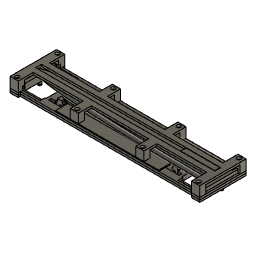
Switch blade (Autodesk Fusion 360 design; units mm, degrees)
Autodesk Fusion 360 part; units mm, degrees
note: some values were not read from the file. Chosen so that the rebuilt part matches the saved one: which bodies a step acts on; which face or edge a step refers to. Set by a fixed rule: which sketch regions a step uses.
(part 1 of 2)
sketch "base" plane through (0, 0, 0) normal (0, 0, 1) x (1, 0, 0)
  line L0 (0, 0) -> (180, 0)
  line L1 (180, 0) -> (180, 40)
  line L2 (180, 40) -> (0, 40)
  line L3 (0, 40) -> (0, 0)
  dimension "d3" = 40
  dimension "d4" = 180
  constraint horizontal L0
  constraint vertical L1
  constraint horizontal L2
  constraint vertical L3
  constraint coincident L0.start L3.end
  measures "d3" distance of L0.start L2.end
  measures "d4" distance of L0.start L0.end
ref_plane "WorkPlane1" through (90, 20, 2) normal (0, 0, 1) x (1, 0, 0)
sketch "catchCutout" plane through (0, 0, 2) normal (0, 0, 1) x (1, 0, 0)
  line L0 (147.75, 33.25) -> (144.75, 33.25)
  line L1 (144.75, 33.25) -> (144.75, 10)
  line L2 (144.75, 10) -> (147.75, 10)
  line L3 (147.75, 10) -> (147.75, 33.25)
  line L4 (144.5, 33.5) -> (148, 33.5)
  line L5 (148, 33.5) -> (148, 6.5)
  line L6 (148, 6.5) -> (144.5, 6.5)
  line L7 (144.5, 6.5) -> (144.5, 33.5)
  line L8 (150, 0) -> (150, 40)
  line L9 (0, 0) -> (150, 0)
  line L10 (150, 40) -> (0, 40)
  line L11 (144.75, 10) -> (141.75, 10)
  line L12 (141.75, 10) -> (141.75, 14)
  line L13 (141.75, 14) -> (144.75, 14)
  line L14 (144.75, 14) -> (144.75, 10)
  line L15 (144.5, 6.5) -> (125.5, 6.5)
  line L16 (125.5, 6.5) -> (125.5, 14.25)
  line L17 (125.5, 14.25) -> (144.5, 14.25)
  line L18 (144.5, 14.25) -> (144.5, 6.5)
  circle A0 centre (128.5, 9.5) radius 2.5
  line L19 (90, 40) -> (90, 0)
  line L20 (144.5, 18.0289) -> (148, 18.0289)
  line L21 (147.75, 10) -> (151.75, 10)
  line L22 (151.75, 10) -> (151.75, 12)
  line L23 (151.75, 12) -> (147.75, 12)
  line L24 (147.75, 12) -> (147.75, 10)
  line L25 (148, 6.5) -> (152, 6.5)
  line L26 (152, 6.5) -> (152, 9)
  line L27 (152, 9) -> (148, 9)
  line L28 (148, 9) -> (148, 6.5)
  line L29 (152, 9) -> (148, 9)
  line L30 (148, 9) -> (148, 12.25)
  line L31 (148, 12.25) -> (152, 12.25)
  line L32 (152, 12.25) -> (152, 9)
  line L33 (144.75, 33.25) -> (140.75, 33.25)
  line L34 (140.75, 33.25) -> (140.75, 31.25)
  line L35 (140.75, 31.25) -> (144.75, 31.25)
  line L36 (144.75, 31.25) -> (144.75, 33.25)
  line L37 (144.5, 33.5) -> (140.5, 33.5)
  line L38 (140.5, 33.5) -> (140.5, 30.25)
  line L39 (140.5, 30.25) -> (144.5, 30.25)
  line L40 (144.5, 30.25) -> (144.5, 33.5)
  line L41 (140.5, 30.25) -> (144.5, 30.25)
  line L42 (144.5, 30.25) -> (144.5, 27.75)
  line L43 (144.5, 27.75) -> (140.5, 27.75)
  line L44 (140.5, 27.75) -> (140.5, 30.25)
  line L45 (147.75, 12) -> (139.7117, 12)
  line L46 (144.5, 27.75) -> (148, 27.75)
  line L47 (144.75, 31.25) -> (147.75, 31.25)
  line L48 (35.25, 31.25) -> (35.25, 33.25)
  line L49 (28, 12.25) -> (28, 9)
  line L50 (39.5, 27.75) -> (39.5, 30.25)
  line L51 (32.25, 10) -> (28.25, 10)
  line L52 (35.5, 18.0289) -> (32, 18.0289)
  line L53 (38.25, 10) -> (38.25, 14)
  line L54 (35.25, 33.25) -> (35.25, 10)
  line L55 (32.25, 10) -> (32.25, 33.25)
  line L56 (35.5, 6.5) -> (35.5, 33.5)
  line L57 (28.25, 10) -> (28.25, 12)
  line L58 (32, 12.25) -> (28, 12.25)
  line L59 (38.25, 14) -> (35.25, 14)
  line L60 (54.5, 14.25) -> (35.5, 14.25)
  line L61 (32, 9) -> (32, 12.25)
  circle A1 centre (51.5, 9.5) radius 2.5
  line L62 (28.25, 12) -> (32.25, 12)
  line L63 (32, 33.5) -> (32, 6.5)
  line L64 (32.25, 12) -> (40.2883, 12)
  line L65 (28, 6.5) -> (28, 9)
  line L66 (35.25, 10) -> (32.25, 10)
  line L67 (35.25, 14) -> (35.25, 10)
  line L68 (32, 6.5) -> (35.5, 6.5)
  line L69 (35.25, 33.25) -> (39.25, 33.25)
  line L70 (32, 9) -> (32, 6.5)
  line L71 (35.5, 27.75) -> (32, 27.75)
  line L72 (35.25, 10) -> (38.25, 10)
  line L73 (28, 9) -> (32, 9)
  line L74 (39.25, 33.25) -> (39.25, 31.25)
  line L75 (32.25, 12) -> (32.25, 10)
  line L76 (35.5, 33.5) -> (39.5, 33.5)
  line L77 (39.25, 31.25) -> (35.25, 31.25)
  line L78 (32.25, 33.25) -> (35.25, 33.25)
  line L79 (35.5, 27.75) -> (39.5, 27.75)
  line L80 (39.5, 30.25) -> (35.5, 30.25)
  line L81 (35.5, 14.25) -> (35.5, 6.5)
  line L82 (35.25, 31.25) -> (32.25, 31.25)
  line L83 (39.5, 30.25) -> (35.5, 30.25)
  line L84 (28, 9) -> (32, 9)
  line L85 (35.5, 30.25) -> (35.5, 33.5)
  line L86 (32, 6.5) -> (28, 6.5)
  line L87 (35.5, 30.25) -> (35.5, 27.75)
  line L88 (35.5, 6.5) -> (54.5, 6.5)
  line L89 (54.5, 6.5) -> (54.5, 14.25)
  line L90 (35.5, 33.5) -> (32, 33.5)
  line L91 (39.5, 33.5) -> (39.5, 30.25)
  line L92 (180, 0) -> (180, 40)
  line L93 (180, 40) -> (0, 40)
  line L94 (0, 0) -> (180, 0)
  point P0 (90, 40)
  dimension "d12" = 6.5
  dimension "d13" = 6.5
  dimension "d14" = 0.25
  dimension "d15" = 0.25
  dimension "d17" = 0.25
  dimension "d18" = 3.5
  dimension "d20" = 19
  dimension "d21" = 3.5
  dimension "d22" = 4
  dimension "d23" = 7.75
  dimension "d24" = 3
  dimension "d25" = 5
  dimension "d26" = 3
  dimension "d27" = 3
  dimension "d36" = 3
  dimension "d88" = 4
  dimension "d89" = 2
  dimension "d90" = 4
  dimension "d91" = 2.5
  dimension "d92" = 0.25
  dimension "d94" = 4
  dimension "d95" = 2
  dimension "d96" = 0.25
  dimension "d97" = 2.5
  dimension "d98" = 3.5
  dimension "d303" = 32
  constraint horizontal L0
  constraint vertical L1
  constraint horizontal L2
  constraint vertical L3
  constraint horizontal L4
  constraint vertical L5
  constraint horizontal L6
  constraint vertical L7
  constraint horizontal L11
  constraint vertical L12
  constraint horizontal L13
  constraint vertical L14
  constraint coincident L1 L2.start
  constraint horizontal L15
  constraint vertical L16
  constraint horizontal L17
  constraint vertical L18
  constraint coincident L10 P0
  constraint coincident P0 L19.start
  constraint coincident L7 L20.start
  constraint coincident L5 L20.end
  constraint perpendicular L5 L20
  constraint horizontal L21
  constraint vertical L22
  constraint horizontal L23
  constraint vertical L24
  constraint horizontal L25
  constraint vertical L26
  constraint horizontal L27
  constraint vertical L28
  constraint horizontal L29
  constraint vertical L30
  constraint horizontal L31
  constraint vertical L32
  constraint coincident L5 L30.end
  constraint horizontal L33
  constraint vertical L34
  constraint horizontal L35
  constraint vertical L36
  constraint horizontal L37
  constraint vertical L38
  constraint horizontal L39
  constraint vertical L40
  constraint horizontal L41
  constraint vertical L42
  constraint horizontal L43
  constraint vertical L44
  constraint coincident L7 L42.end
  constraint perpendicular L3 L45
  constraint coincident L5 L46.end
  constraint perpendicular L5 L46
  constraint coincident L3 L47.end
  constraint perpendicular L3 L47
  constraint symmetric L0.start L19 L55.end
  constraint symmetric L0.end L19 L48.end
  constraint symmetric L1.end L19 L54.end
  constraint symmetric L2.end L19 L51.start
  constraint symmetric L4.start L19 L56.end
  constraint symmetric L4.end L19 L63.start
  constraint symmetric L5.end L19 L63.end
  constraint symmetric L6.end L19 L56.start
  constraint symmetric L11.end L19 L53.start
  constraint symmetric L12.end L19 L53.end
  constraint symmetric L13.end L19 L59.end
  constraint symmetric L15.end L19 L88.end
  constraint symmetric L16.end L19 L60.start
  constraint symmetric L17.end L19 L60.end
  constraint symmetric A0 L19 A1
  constraint symmetric L19 L20.start L52.start
  constraint symmetric L19 L20.end L52.end
  constraint symmetric L19 L21.end L51.end
  constraint symmetric L19 L22.end L57.end
  constraint symmetric L19 L23.end L62.end
  constraint symmetric L19 L25.end L65.start
  constraint symmetric L19 L26.end L49.end
  constraint symmetric L19 L27.end L61.start
  constraint symmetric L19 L30.end L58.start
  constraint symmetric L19 L31.end L49.start
  constraint symmetric L19 L33.end L69.end
  constraint symmetric L19 L34.end L74.end
  constraint symmetric L19 L35.end L48.start
  constraint symmetric L19 L37.end L76.end
  constraint symmetric L19 L38.end L50.end
  constraint symmetric L19 L39.end L80.end
  constraint symmetric L19 L42.end L71.start
  constraint symmetric L19 L43.end L50.start
  constraint symmetric L19 L45.end L64.end
  constraint symmetric L19 L46.end L71.end
  constraint symmetric L19 L47.end L82.end
  constraint midpoint P0 L93
  constraint midpoint L19.end L94
  measures "d12" distance of L6 L9
  measures "d13" distance of L4 L10
  measures "d14" distance of L3 L5
  measures "d15" distance of L1 L7
  measures "d17" distance of L0 L4
  measures "d18" distance of L2 L6
  measures "d20" distance of L6.end L15.end
  measures "d21" distance of L11 L15
  measures "d22" distance of L11.end L12.end
  measures "d23" distance of L15.end L16.end
  measures "d24" distance of L15 A0.centre
  measures "d25" diameter of A0
  measures "d26" distance of L16 A0.centre
  measures "d27" distance of L1 L12
  measures "d36" distance of L1 L3
  measures "d88" distance of L2.end L22
  measures "d89" distance of L21.end L22.end
  measures "d90" distance of L5.end L25.end
  measures "d91" distance of L25.end L26.end
  measures "d92" distance of L23 L31
  measures "d94" distance of L0.end L33.end
  measures "d95" distance of L33.end L34.end
  measures "d96" distance of L34 L38
  measures "d97" distance of L39 L43
  measures "d98" distance of L35 L43
  measures "d303" distance of L5 L92
sketch "puller" plane through (75, 20, 2) normal (0, 0, 1) x (1, 0, 0)
  line L0 (102.75, 16.25) -> (82, 16.25)
  line L1 (82, -16.25) -> (102.75, -16.25)
  line L2 (102.75, -16.25) -> (102.75, 16.25)
  line L3 (82, 16.25) -> (74.75, 16.25)
  line L4 (74.75, 16.25) -> (74.75, 13.75)
  line L5 (74.75, 13.75) -> (99.75, 13.75)
  line L6 (82, -16.25) -> (74.75, -16.25)
  line L7 (74.75, -16.25) -> (74.75, -13.75)
  line L8 (74.75, -13.75) -> (99.75, -13.75)
  line L9 (99.75, 13.75) -> (99.75, -13.75)
  line L10 (103, 16.5) -> (54.5, 16.5)
  line L11 (54.5, 16.5) -> (54.5, 13.5)
  line L12 (54.5, 13.5) -> (79.5, 13.5)
  line L13 (79.5, 13.5) -> (79.5, -13.5)
  line L14 (79.5, -13.5) -> (54.5, -13.5)
  line L15 (54.5, -13.5) -> (54.5, -16.5)
  line L16 (54.5, -16.5) -> (103, -16.5)
  line L17 (103, -16.5) -> (103, 16.5)
  line L18 (99.75, -13.75) -> (102.75, -13.75)
  line L19 (99.75, 13.75) -> (102.75, 13.75)
  line L20 (105, -20) -> (105, 20)
  line L21 (-75, -20) -> (105, -20)
  line L22 (105, 20) -> (-75, 20)
  line L23 (102.75, 0) -> (102.75, -13.25)
  line L24 (102.75, 0) -> (102.75, 13.25)
  line L25 (102.75, 13.25) -> (79.5, 13.25)
  line L26 (102.75, -13.25) -> (79.5, -13.25)
  line L27 (79.5, -13.5) -> (102.75, -13.5)
  line L28 (79.5, 13.5) -> (102.75, 13.5)
  line L29 (102.75, -16.25) -> (100.75, -16.25)
  line L30 (100.75, -16.25) -> (100.75, -17.75)
  line L31 (100.75, -17.75) -> (102.75, -17.75)
  line L32 (102.75, -17.75) -> (102.75, -16.25)
  line L33 (103, -16.5) -> (100.5, -16.5)
  line L34 (100.5, -16.5) -> (100.5, -18)
  line L35 (100.5, -18) -> (103, -18)
  line L36 (103, -18) -> (103, -16.5)
  line L37 (100.5, -18) -> (80.5, -18)
  line L38 (80.5, -18) -> (80.5, -16.5)
  line L39 (80.5, -16.5) -> (100.5, -16.5)
  line L40 (100.5, -16.5) -> (100.5, -18)
  line L41 (102.75, 16.25) -> (100.75, 16.25)
  line L42 (100.75, 16.25) -> (100.75, 17.75)
  line L43 (100.75, 17.75) -> (102.75, 17.75)
  line L44 (102.75, 17.75) -> (102.75, 16.25)
  line L45 (103, 16.5) -> (100.5, 16.5)
  line L46 (100.5, 16.5) -> (100.5, 18)
  line L47 (100.5, 18) -> (103, 18)
  line L48 (103, 18) -> (103, 16.5)
  line L49 (100.5, 18) -> (80.5, 18)
  line L50 (80.5, 18) -> (80.5, 16.5)
  line L51 (80.5, 16.5) -> (100.5, 16.5)
  line L52 (100.5, 16.5) -> (100.5, 18)
  line L53 (100.75, -16.25) -> (100.75, -13.25)
  line L54 (80.5, -16.5) -> (80.5, -13.25)
  line L55 (100.75, 16.25) -> (100.75, 13.25)
  line L56 (80.5, 16.5) -> (80.5, 13.25)
  line L57 (15, 20) -> (15, -20)
  line L58 (-70.75, 17.75) -> (-72.75, 17.75)
  line L59 (-73, -16.5) -> (-70.5, -16.5)
  line L60 (-69.75, 13.75) -> (-72.75, 13.75)
  line L61 (-70.75, -17.75) -> (-72.75, -17.75)
  line L62 (-73, -18) -> (-73, -16.5)
  line L63 (-72.75, 17.75) -> (-72.75, 16.25)
  line L64 (-73, 16.5) -> (-24.5, 16.5)
  line L65 (-52, -16.25) -> (-72.75, -16.25)
  line L66 (-49.5, -13.5) -> (-72.75, -13.5)
  line L67 (-44.75, -16.25) -> (-44.75, -13.75)
  line L68 (-72.75, -17.75) -> (-72.75, -16.25)
  line L69 (-70.75, -16.25) -> (-70.75, -17.75)
  line L70 (-50.5, 16.5) -> (-70.5, 16.5)
  line L71 (-44.75, 16.25) -> (-44.75, 13.75)
  line L72 (-24.5, -13.5) -> (-24.5, -16.5)
  line L73 (-49.5, 13.5) -> (-72.75, 13.5)
  line L74 (-50.5, -16.5) -> (-70.5, -16.5)
  line L75 (-44.75, 13.75) -> (-69.75, 13.75)
  line L76 (-44.75, -13.75) -> (-69.75, -13.75)
  line L77 (-70.5, -16.5) -> (-70.5, -18)
  line L78 (-70.5, 18) -> (-73, 18)
  line L79 (-72.75, -13.25) -> (-49.5, -13.25)
  line L80 (-50.5, -18) -> (-50.5, -16.5)
  line L81 (-72.75, -16.25) -> (-70.75, -16.25)
  line L82 (-24.5, 13.5) -> (-49.5, 13.5)
  line L83 (-52, -16.25) -> (-44.75, -16.25)
  line L84 (-72.75, 16.25) -> (-52, 16.25)
  line L85 (-72.75, 13.25) -> (-49.5, 13.25)
  line L86 (-50.5, 16.5) -> (-50.5, 13.25)
  line L87 (-50.5, 18) -> (-50.5, 16.5)
  line L88 (-70.75, 16.25) -> (-70.75, 17.75)
  line L89 (-70.5, 18) -> (-50.5, 18)
  line L90 (-73, 16.5) -> (-70.5, 16.5)
  line L91 (-73, 18) -> (-73, 16.5)
  line L92 (-52, 16.25) -> (-44.75, 16.25)
  line L93 (-24.5, 16.5) -> (-24.5, 13.5)
  line L94 (-70.5, 16.5) -> (-70.5, 18)
  line L95 (-24.5, -16.5) -> (-73, -16.5)
  line L96 (-70.75, 16.25) -> (-70.75, 13.25)
  line L97 (-50.5, -16.5) -> (-50.5, -13.25)
  line L98 (-72.75, 0) -> (-72.75, -13.25)
  line L99 (-70.5, 16.5) -> (-70.5, 18)
  line L100 (-70.5, -18) -> (-73, -18)
  line L101 (-72.75, 16.25) -> (-70.75, 16.25)
  line L102 (-49.5, -13.5) -> (-24.5, -13.5)
  line L103 (-70.75, -16.25) -> (-70.75, -13.25)
  line L104 (-69.75, 13.75) -> (-69.75, -13.75)
  line L105 (-72.75, -16.25) -> (-72.75, 16.25)
  line L106 (-70.5, -16.5) -> (-70.5, -18)
  line L107 (-73, -16.5) -> (-73, 16.5)
  line L108 (-72.75, 0) -> (-72.75, 13.25)
  line L109 (-69.75, -13.75) -> (-72.75, -13.75)
  line L110 (-49.5, 13.5) -> (-49.5, -13.5)
  line L111 (-70.5, -18) -> (-50.5, -18)
  point P0 (105, 0)
  dimension "d39" = 2
  dimension "d40" = 3.5
  dimension "d41" = 3.5
  dimension "d42" = 0.25
  dimension "d43" = 0.25
  dimension "d44" = 0.25
  dimension "d45" = 0.25
  dimension "d46" = 0.25
  dimension "d47" = 3
  dimension "d48" = 3
  dimension "d49" = 25
  dimension "d50" = 3
  dimension "d51" = 25
  dimension "d52" = 20.25
  dimension "d53" = 20.25
  dimension "d54" = 20.25
  dimension "d74" = 0.25
  dimension "d136" = 2
  dimension "d137" = 1.5
  dimension "d138" = 2.5
  dimension "d139" = 1.5
  dimension "d140" = 20
  dimension "d141" = 2
  dimension "d142" = 1.5
  dimension "d143" = 2.5
  dimension "d144" = 1.5
  dimension "d145" = 20
  constraint horizontal L0
  constraint horizontal L1
  constraint vertical L2
  constraint horizontal L3
  constraint vertical L4
  constraint horizontal L5
  constraint horizontal L6
  constraint vertical L7
  constraint horizontal L8
  constraint perpendicular L8 L9
  constraint perpendicular L2 L10
  constraint perpendicular L10 L11
  constraint perpendicular L11 L12
  constraint perpendicular L10 L13
  constraint perpendicular L13 L14
  constraint perpendicular L14 L15
  constraint perpendicular L15 L16
  constraint perpendicular L10 L17
  constraint coincident L2 L18.end
  constraint perpendicular L2 L18
  constraint coincident L2 L19.end
  constraint perpendicular L2 L19
  constraint midpoint L20 P0
  constraint midpoint L2 L23.start
  constraint coincident L2 L23.end
  constraint parallel L2 L23
  constraint coincident L2 L24.end
  constraint parallel L2 L24
  constraint equal L23 L24
  constraint coincident L13 L25.end
  constraint perpendicular L13 L25
  constraint coincident L13 L26.end
  constraint perpendicular L13 L26
  constraint coincident L2 L27.end
  constraint perpendicular L2 L27
  constraint coincident L2 L28.end
  constraint perpendicular L2 L28
  constraint horizontal L29
  constraint vertical L30
  constraint horizontal L31
  constraint vertical L32
  constraint horizontal L33
  constraint vertical L34
  constraint horizontal L35
  constraint vertical L36
  constraint horizontal L37
  constraint vertical L38
  constraint horizontal L39
  constraint vertical L40
  constraint coincident L16 L38.end
  constraint horizontal L41
  constraint vertical L42
  constraint horizontal L43
  constraint vertical L44
  constraint horizontal L45
  constraint vertical L46
  constraint horizontal L47
  constraint vertical L48
  constraint horizontal L49
  constraint vertical L50
  constraint horizontal L51
  constraint vertical L52
  constraint coincident L26 L53.end
  constraint perpendicular L26 L53
  constraint coincident L26 L54.end
  constraint perpendicular L26 L54
  constraint coincident L25 L55.end
  constraint perpendicular L25 L55
  constraint coincident L25 L56.end
  constraint perpendicular L25 L56
  constraint midpoint L22 L57.start
  constraint midpoint L21 L57.end
  constraint symmetric L0.start L57 L63.end
  constraint symmetric L0.end L57 L84.end
  constraint symmetric L1.start L57 L65.start
  constraint symmetric L1.end L57 L65.end
  constraint symmetric L3.end L57 L71.start
  constraint symmetric L4.end L57 L71.end
  constraint symmetric L5.end L57 L60.start
  constraint symmetric L6.end L57 L67.start
  constraint symmetric L7.end L57 L67.end
  constraint symmetric L8.end L57 L76.end
  constraint symmetric L10.start L57 L64.start
  constraint symmetric L10.end L57 L64.end
  constraint symmetric L11.end L57 L82.start
  constraint symmetric L12.end L57 L73.start
  constraint symmetric L13.end L57 L66.start
  constraint symmetric L14.end L57 L72.start
  constraint symmetric L15.end L57 L72.end
  constraint symmetric L16.end L57 L59.start
  constraint symmetric L18.end L57 L109.end
  constraint symmetric L19.end L57 L60.end
  constraint symmetric L23.start L57 L98.start
  constraint symmetric L23.end L57 L79.start
  constraint symmetric L24.end L57 L85.start
  constraint symmetric L25.end L57 L85.end
  constraint symmetric L26.end L57 L79.end
  constraint symmetric L27.end L57 L66.end
  constraint symmetric L28.end L57 L73.end
  constraint symmetric L29.end L57 L69.start
  constraint symmetric L30.end L57 L61.start
  constraint symmetric L31.end L57 L61.end
  constraint symmetric L33.end L57 L59.end
  constraint symmetric L34.end L57 L77.end
  constraint symmetric L35.end L57 L62.start
  constraint symmetric L37.end L57 L80.start
  constraint symmetric L38.end L57 L74.start
  constraint symmetric L41.end L57 L88.start
  constraint symmetric L42.end L57 L58.start
  constraint symmetric L43.end L57 L58.end
  constraint symmetric L45.end L57 L70.end
  constraint symmetric L46.end L57 L78.start
  constraint symmetric L47.end L57 L78.end
  constraint symmetric L49.end L57 L87.start
  constraint symmetric L50.end L57 L70.start
  constraint symmetric L53.end L57 L103.end
  constraint symmetric L54.end L57 L97.end
  constraint symmetric L55.end L57 L96.end
  constraint symmetric L56.end L57 L86.end
  measures "d39" distance of L17 L20
  measures "d40" distance of L16 L21
  measures "d41" distance of L10 L22
  measures "d42" distance of L6 L16
  measures "d43" distance of L3 L10
  measures "d44" distance of L2 L17
  measures "d45" distance of L5 L12
  measures "d46" distance of L8 L14
  measures "d47" distance of L10 L12
  measures "d48" distance of L14 L16
  measures "d49" distance of L4 L9
  measures "d50" distance of L2 L9
  measures "d51" distance of L7 L9
  measures "d52" distance of L9 L13
  measures "d53" distance of L4 L11
  measures "d54" distance of L7 L15
  measures "d74" distance of L14 L26
  measures "d136" distance of L1.end L29.end
  measures "d137" distance of L1.end L31.end
  measures "d138" distance of L34.end L35.end
  measures "d139" distance of L16.end L35.end
  measures "d140" distance of L34.end L37.end
  measures "d141" distance of L0.start L41.end
  measures "d142" distance of L0.start L43.end
  measures "d143" distance of L10.start L45.end
  measures "d144" distance of L10.start L47.end
  measures "d145" distance of L46.end L49.end
sketch "slide" plane through (75, 20, 2) normal (0, 0, 1) x (1, 0, 0)
  line L0 (105, -20) -> (105, 20)
  line L1 (105, 0) -> (105, 4.4885)
  line L2 (105, 0) -> (105, -4.4885)
  line L3 (105, 4.4885) -> (99.5, 4.4885)
  line L4 (99.5, 4.4885) -> (-49.5, 4.4885)
  line L5 (105, -4.4885) -> (-49.5, -4.4885)
  line L6 (-49.5, -4.4885) -> (-49.5, 4.4885)
  line L7 (99.5, 4.4885) -> (99.5, -4.4885)
  line L8 (69, -2.2385) -> (69, -4.4885)
  line L9 (92.5, 4.4885) -> (92.5, -4.4885)
  line L10 (69, -2.2385) -> (92.5, -2.2385)
  line L11 (75, -20) -> (75, 20)
  line L12 (99.75, 4.7385) -> (-69.75, 4.7385)
  line L13 (-69.75, 4.7385) -> (-69.75, -4.7385)
  line L14 (-69.75, -4.7385) -> (99.75, -4.7385)
  line L15 (99.75, -4.7385) -> (99.75, 4.7385)
  line L16 (72.75, -10) -> (72.75, 13.25)
  line L17 (66.75, 4.4885) -> (69.75, 4.4885)
  line L18 (92.5, -4.4885) -> (90.25, -2.2385)
  line L19 (74.1958, -4.4885) -> (72.75, -4.4885)
  line L20 (72.75, -4.4885) -> (72.75, -2.4885)
  line L21 (41.75, -4.4885) -> (38.75, -4.4885)
  line L22 (38.75, -4.4885) -> (38.75, -7.4885)
  line L23 (38.75, -7.4885) -> (41.75, -7.4885)
  line L24 (41.75, -7.4885) -> (41.75, -4.4885)
  line L25 (41.75, -4.4885) -> (41.75, 4.4885)
  line L26 (41.75, 4.4885) -> (38.75, 4.4885)
  line L27 (38.75, 4.4885) -> (38.75, 7.4885)
  line L28 (38.75, 7.4885) -> (41.75, 7.4885)
  line L29 (41.75, 7.4885) -> (41.75, 4.4885)
  line L30 (45, -4.7385) -> (41.5, -4.7385)
  line L31 (41.5, -4.7385) -> (41.5, -7.7385)
  line L32 (41.5, -7.7385) -> (45, -7.7385)
  line L33 (45, -7.7385) -> (45, -4.7385)
  line L34 (41.5, -7.7385) -> (18.5, -7.7385)
  line L35 (18.5, -7.7385) -> (18.5, -5.0528)
  line L36 (18.5, -5.0528) -> (41.5, -5.0528)
  line L37 (41.5, -5.0528) -> (41.5, -7.7385)
  line L38 (18.5, -5.0528) -> (18.5, 4.7385)
  line L39 (45, -4.7385) -> (45, 4.7385)
  line L40 (45, 4.7385) -> (41.5, 4.7385)
  line L41 (41.5, 4.7385) -> (41.5, 7.7385)
  line L42 (41.5, 7.7385) -> (45, 7.7385)
  line L43 (45, 7.7385) -> (45, 4.7385)
  line L44 (41.5, 7.7385) -> (18.5, 7.7385)
  line L45 (18.5, 7.7385) -> (18.5, 4.7385)
  line L46 (18.5, 4.7385) -> (41.5, 4.7385)
  line L47 (41.5, 4.7385) -> (41.5, 7.7385)
  line L48 (41.5, 4.7385) -> (41.5, -4.7385)
  line L49 (38.75, -4.4885) -> (38.75, 4.4885)
  line L50 (69.75, -6) -> (69.75, -10)
  line L51 (69.75, 13.25) -> (69.75, -10)
  line L52 (69.75, -10) -> (72.75, -10)
  line L53 (-75, 20) -> (-75, -20)
  line L54 (25, 4.4885) -> (25, -4.4885)
  line L55 (-49.5, 4.4885) -> (99.5, 4.4885)
  line L56 (-19.75, -6) -> (-19.75, -10)
  line L57 (-42.5, 4.4885) -> (-42.5, -4.4885)
  line L58 (-22.75, -10) -> (-22.75, 13.25)
  line L59 (-19, -2.2385) -> (-42.5, -2.2385)
  line L60 (-42.5, -4.4885) -> (-40.25, -2.2385)
  line L61 (-19.75, 13.25) -> (-19.75, -10)
  line L62 (-22.75, -4.4885) -> (-22.75, -2.4885)
  line L63 (-22.75, -2.4885) -> (-24.9574, -2.4584)
  line L64 (-16.75, 4.4885) -> (-19.75, 4.4885)
  line L65 (-24.9574, -2.4584) -> (-24.1958, -4.4885)
  line L66 (-19.75, -10) -> (-22.75, -10)
  line L67 (-24.1958, -4.4885) -> (-22.75, -4.4885)
  line L68 (-19, -2.2385) -> (-19, -4.4885)
  line L69 (-49.75, 4.7385) -> (119.75, 4.7385)
  line L70 (-55, -4.4885) -> (99.5, -4.4885)
  line L71 (119.75, -4.7385) -> (-49.75, -4.7385)
  line L72 (-42.75, -10) -> (-42.75, 13.25)
  line L73 (-39.75, 13.25) -> (-39.75, -10)
  line L74 (-39.75, -10) -> (-42.75, -10)
  line L75 (-22.75, -2.4885) -> (-42.75, -2.4885)
  line L76 (72.75, -2.4885) -> (69.75, -2.4885)
  line L77 (105, -20) -> (105, 20)
  point P0 (105, 0)
  point P1 (25, 4.4885)
  dimension "d56" = 5.5
  dimension "d60" = 23.5
  dimension "d63" = 0.25
  dimension "d64" = 0.25
  dimension "d65" = 0.25
  dimension "d66" = 20.25
  dimension "d67" = 45
  dimension "d69" = 2.25
  dimension "d146" = 3
  dimension "d147" = 3
  dimension "d148" = 3
  dimension "d149" = 3
  dimension "d150" = 3.5
  dimension "d151" = 3
  dimension "d152" = 3.25
  dimension "d153" = 23
  dimension "d154" = 3.5
  dimension "d155" = 3
  dimension "d157" = 24
  dimension "d259" = 5.25
  dimension "d277" = 74.5
  dimension "d278" = 74.5
  dimension "d302" = 2
  dimension "d304" = 12.5
  constraint midpoint P0 L0
  constraint coincident P0 L1.start
  constraint coincident L0 L1.end
  constraint coincident L0 L2.end
  constraint equal L1 L2
  constraint perpendicular L0 L3
  constraint perpendicular L0 L4
  constraint perpendicular L2 L5
  constraint perpendicular L4 L6
  constraint coincident L4 L3.end
  constraint coincident L5 L7.end
  constraint perpendicular L5 L7
  constraint perpendicular L4 L8
  constraint coincident L4 L9.start
  constraint coincident L5 L9.end
  constraint perpendicular L5 L9
  constraint perpendicular L9 L10
  constraint coincident L9 L10.end
  constraint horizontal L12
  constraint vertical L13
  constraint horizontal L14
  constraint vertical L15
  constraint horizontal L17
  constraint coincident L4 L17.start
  constraint coincident L5 L8.end
  constraint coincident L10 L18.end
  constraint horizontal L19
  constraint vertical L20
  constraint coincident L16 L20.end
  constraint coincident L5 L19.start
  constraint horizontal L21
  constraint vertical L22
  constraint horizontal L23
  constraint vertical L24
  constraint coincident L5 L21.start
  constraint coincident L4 L25.end
  constraint perpendicular L4 L25
  constraint horizontal L26
  constraint vertical L27
  constraint horizontal L28
  constraint vertical L29
  constraint horizontal L30
  constraint vertical L31
  constraint horizontal L32
  constraint vertical L33
  constraint coincident L14 L30.start
  constraint horizontal L34
  constraint vertical L35
  constraint horizontal L36
  constraint vertical L37
  constraint coincident L12 L38.end
  constraint perpendicular L12 L38
  constraint coincident L12 L39.end
  constraint perpendicular L12 L39
  constraint horizontal L40
  constraint vertical L41
  constraint horizontal L42
  constraint vertical L43
  constraint horizontal L44
  constraint vertical L45
  constraint horizontal L46
  constraint vertical L47
  constraint midpoint L4 P1
  constraint coincident P1 L54.start
  constraint coincident L5 L54.end
  constraint perpendicular L5 L54
  constraint symmetric L2.end L54 L70.start
  constraint symmetric L3.end L54 L4.end
  constraint symmetric L4.end L54 L3.end
  constraint symmetric L5.end L54 L7.end
  constraint symmetric L8.start L54 L59.start
  constraint symmetric L8.end L54 L68.end
  constraint symmetric L9.start L54 L57.start
  constraint symmetric L9.end L54 L57.end
  constraint symmetric L10.end L54 L59.end
  constraint symmetric L12.start L54 L69.start
  constraint symmetric L12.end L54 L69.end
  constraint symmetric L13.end L54 L71.start
  constraint symmetric L14.end L54 L71.end
  constraint symmetric L16.start L54 L58.start
  constraint symmetric L16.end L54 L58.end
  constraint symmetric L17.start L54 L64.start
  constraint symmetric L17.end L54 L64.end
  constraint symmetric L18.end L54 L60.end
  constraint symmetric L19.start L54 L65.end
  constraint symmetric L19.end L54 L62.start
  constraint symmetric L20.end L54 L62.end
  constraint symmetric L50.start L54 L56.start
  constraint symmetric L50.end L54 L56.end
  constraint symmetric L51.start L54 L61.start
  constraint coincident L72 L75.end
  constraint perpendicular L72 L75
  constraint coincident L51 L76.end
  constraint perpendicular L51 L76
  measures "d56" distance of L1 L7
  measures "d60" distance of L8 L9
  measures "d63" distance of L4 L12
  measures "d64" distance of L5 L14
  measures "d65" distance of L7 L15
  measures "d66" distance of L6 L13
  measures "d67" angle of L9 L18
  measures "d69" distance of L5 L10
  measures "d146" distance of L21.start L21.end
  measures "d147" distance of L21.start L23.end
  measures "d148" distance of L25.end L26.end
  measures "d149" distance of L25.end L28.end
  measures "d150" distance of L30.start L30.end
  measures "d151" distance of L30.start L32.end
  measures "d152" distance of L24 L33
  measures "d153" distance of L31.end L34.end
  measures "d154" distance of L39.end L40.end
  measures "d155" distance of L39.end L42.end
  measures "d157" distance of L8 L39
  measures "d259" distance of L13 L53
  measures "d277" distance of L4.end P1
  measures "d278" distance of L3.end P1
  measures "d302" distance of L70 L76
  measures "d304" distance of L9 L77
extrude "base (1)" add sketch "base" along normal blind 4 makes body 1
extrude "topCutout" cut sketch "puller" sketch "catchCutout" sketch "slide" along normal blind 4.5 contours L0 L2 L19 L41 L55 | L2 L10 L16 L17 L23 L24 L32 L33 L44 L45 | L0 L10 L41 L42 L44 L45 | L0 L3 L5 L19 L55 L56 | L0 L3 L10 L42 L45 L51 L56 | L2 L19 L28 L55 | L10 L42 L43 L44 L45 L46 L47 L48 L52 | L10 L42 L43 L44 L45 | L9 L19 L28 L55 | L2 L25 L28 L55 | L10 L46 L49 L50 L51 L52 | L5 L9 L28 L56 | L9 L25 L28 L55 | L2 L9 L23 L24 L25 L26 | L16 L30 L31 L32 L33 L34 L35 L36 L40 | L9 L25 L28 L56 | L16 L30 L31 L32 L33 | L1 L16 L29 L30 L32 L33 | L13 L25 L28 L56 | L9 L13 L25 L26 | L2 L26 L27 L53 | L1 L6 L16 L30 L33 L39 L54 | L1 L2 L18 L29 L53 | L16 L34 L37 L38 L39 L40 | L9 L26 L27 L53 | L9 L26 L27 L54 | L2 L18 L27 L53 | L1 L6 L8 L18 L53 L54 | L9 L18 L27 L53 | L8 L9 L27 L54 | L13 L26 L27 L54 | L58 L63 L64 L88 L90 | L58 L63 L64 L78 L88 L90 L91 L94 L99 | L63 L64 L84 L88 L90 L101 | L64 L70 L84 L86 L88 L90 L92 | L59 L63 L64 L68 L90 L95 L98 L105 L107 L108 | L64 L70 L87 L89 L94 L99 | L60 L84 L96 L101 L105 | L60 L75 L84 L86 L92 L96 | L60 L73 L96 L105 | L60 L73 L96 L104 | L59 L61 L62 L68 L69 L77 L95 L100 L106 | L73 L75 L86 L104 | L73 L85 L96 L105 | L73 L85 L96 L104 | L59 L65 L68 L69 L81 L95 | L59 L61 L68 L69 L95 | L73 L85 L86 L104 | L79 L85 L98 L104 L105 L108 | L59 L65 L69 L74 L83 L95 L97 | L65 L81 L103 L105 L109 | L74 L77 L80 L95 L106 L111 | L79 L85 L104 L110 | L65 L76 L83 L97 L103 L109 | L66 L103 L105 L109 | L66 L79 L103 L104 | L66 L79 L97 L104 | L66 L79 L103 L105 | L66 L103 L104 L109 | L66 L79 L97 L110 | L66 L76 L97 L104 of sketch 2 contours L0 L1 L3 L36 L47 | L0 L3 L4 L5 L7 L33 L40 L46 | L1 L7 L33 L35 L36 L40 | L1 L3 L46 L47 | L1 L7 L35 L40 L42 L46 | L3 L5 L20 L46 | L1 L3 L20 L46 | L1 L7 L20 L46 | L3 L5 L20 L23 L30 | L1 L3 L14 L20 L45 | L1 L7 L13 L18 L20 | L7 L39 L41 L42 L43 L44 | L3 L5 L21 L23 L24 L30 | L1 L2 L3 L14 L24 L45 | L1 L7 L13 L14 L18 L45 | L2 L5 L6 L7 L11 L18 L21 L28 L30 | L1 L7 L11 L14 L18 L45 | L7 L11 L12 L13 L15 L16 L17 L18 | L7 L12 L13 L18 L45 | L7 L11 L12 L18 L45 | L5 L8 L25 L27 L28 L29 | L8 L25 L26 L27 L29 | L48 L54 L55 L78 L82 | L54 L56 L71 L77 L85 L87 | L48 L54 L56 L69 L77 L85 | L54 L55 L71 L82 | L55 L56 L63 L69 L71 L78 L85 L90 | L52 L54 L56 L71 | L52 L54 L55 L71 | L52 L54 L55 L64 L67 | L52 L54 L56 L59 L81 | L50 L56 L79 L80 L83 L87 | L52 L55 L63 L71 | L52 L55 L61 L62 L63 | L54 L56 L59 L64 L67 L81 | L53 L56 L59 L60 L72 L81 L88 L89 | L54 L55 L64 L66 L67 L75 | L51 L55 L61 L62 L63 L75 | L54 L56 L64 L67 L72 L81 | L53 L56 L59 L64 L81 | L51 L56 L61 L63 L66 L68 L70 L72 L81 | L53 L56 L64 L72 L81 | L63 L65 L70 L73 L84 L86 of sketch 3 contours L14 L23 L24 L30 L31 L32 L33 L37 L71 | L5 L14 L24 L30 L39 L70 L71 | L14 L23 L24 L30 L31 L37 L71 | L5 L14 L21 L24 L30 L48 L70 L71 | L4 L5 L25 L39 L55 L70 | L4 L12 L29 L39 L40 L55 L69 | L12 L28 L29 L40 L41 L42 L43 L47 L69 | L14 L22 L31 L36 L71 | L5 L14 L21 L22 L48 L70 L71 | L4 L5 L21 L25 L26 L48 L55 L70 | L22 L23 L31 L34 L35 L36 L37 | L4 L12 L26 L29 L40 L48 L55 L69 | L12 L28 L29 L40 L41 L47 L69 | L14 L22 L36 L38 L71 | L5 L14 L22 L38 L70 L71 | L22 L23 L31 L36 L37 | L4 L5 L21 L26 L48 L49 L55 L70 | L4 L12 L26 L27 L46 L48 L55 L69 | L12 L27 L28 L41 L46 L47 L69 | L12 L27 L28 L41 L44 L45 L46 L47 L69 | L4 L5 L49 L54 L55 L70 | L4 L12 L27 L38 L46 L55 L69 | L4 L5 L38 L54 L55 L70 bodies 1
extrude "catchTop" add sketch "catchCutout" along normal blind 2 separate body contours L0 L1 L3 L36 L47 | L1 L3 L46 L47 | L1 L3 L20 L46 | L1 L3 L14 L20 L45 | L1 L2 L3 L14 L24 L45 | L1 L7 L13 L14 L18 L45 | L1 L7 L11 L14 L18 L45 | L7 L12 L13 L18 L45 | L7 L11 L12 L18 L45 makes body 2
extrude "catchTop2" add sketch "catchCutout" along normal blind 2 separate body contours L48 L54 L55 L78 L82 | L54 L55 L71 L82 | L52 L54 L55 L71 | L52 L54 L55 L64 L67 | L54 L56 L59 L64 L67 L81 | L54 L55 L64 L66 L67 L75 | L54 L56 L64 L67 L72 L81 | L53 L56 L59 L64 L81 | L53 L56 L64 L72 L81 makes body 3
extrude "catchSlideBump" add sketch "slide" against normal blind 2 contours L14 L16 L50 L51 L52 L71 | L5 L14 L16 L51 L70 L71 | L5 L16 L20 L51 L70 L76 bodies 2
extrude "catchSlideBump2" add sketch "catchCutout" sketch "slide" against normal blind 2 contours L48 L54 L55 L78 L82 | L48 L54 L56 L69 L77 L85 | L56 L69 L74 L77 L85 | L51 L55 L61 L62 L63 L75 | L51 L57 L61 L62 L63 of sketch 2 contours L14 L71 L72 L73 L74 | L5 L14 L70 L71 L72 L73 | L5 L60 L70 L73 L75 | L5 L57 L70 L72 L75 | L57 L60 L75 bodies 3
extrude "catchHooks" add sketch "catchCutout" against normal blind 2 contours L0 L1 L3 L36 L47 | L1 L7 L33 L35 L36 L40 | L7 L33 L34 L35 L40 | L3 L5 L21 L23 L24 L30 | L5 L8 L21 L23 L30 | L8 L21 L22 L23 bodies 2
extrude "slideCatchMargin" cut 1 faces at (145.75, 22.091, 2) along direction (0, 0, 1) blind 0.7 on bodies 2 bodies 2
extrude "Extrude37" cut 1 faces at (33.25, 26.6705, 2) along direction (0, 0, 1) blind 0.7 on bodies 3 bodies 3
chamfer "Chamfer1" distance 0.7 angle 45 1 edges at (141.75, 12, 4) on bodies 2
chamfer "Chamfer3" distance 0.7 angle 45 1 edges at (38.25, 12, 4) on bodies 3
extrude "baseBottomCutout" cut sketch "catchCutout" sketch "puller" sketch "slide" against normal blind 5 contours L0 L1 L3 L36 L47 | L0 L3 L4 L5 L7 L33 L40 L46 | L1 L7 L33 L35 L36 L40 | L1 L3 L46 L47 | L1 L7 L35 L40 L42 L46 | L7 L33 L34 L35 L37 L38 L39 L40 L41 | L7 L33 L34 L35 L40 | L3 L5 L20 L23 L30 | L1 L3 L14 L20 L45 | L1 L7 L13 L18 L20 | L7 L39 L41 L42 L43 L44 | L3 L5 L21 L23 L24 L30 | L1 L2 L3 L14 L24 L45 | L1 L7 L13 L14 L18 L45 | L2 L5 L6 L7 L11 L18 L21 L28 L30 | L5 L8 L21 L23 L30 | L5 L8 L23 L30 L31 | L1 L7 L11 L14 L18 L45 | L5 L8 L21 L27 L29 L30 | L8 L21 L22 L23 | L8 L21 L22 L23 L27 L29 L31 L32 | L5 L8 L25 L27 L28 L29 | L8 L25 L26 L27 L29 | L48 L54 L55 L78 L82 | L54 L56 L71 L77 L85 L87 | L48 L54 L56 L69 L77 L85 | L54 L55 L71 L82 | L55 L56 L63 L69 L71 L78 L85 L90 | L56 L69 L74 L76 L77 L80 L83 L85 L91 | L56 L69 L74 L77 L85 | L52 L54 L55 L64 L67 | L52 L54 L56 L59 L81 | L50 L56 L79 L80 L83 L87 | L52 L55 L61 L62 L63 | L54 L56 L59 L64 L67 L81 | L54 L55 L64 L66 L67 L75 | L51 L55 L61 L62 L63 L75 | L54 L56 L64 L67 L72 L81 | L49 L51 L57 L58 L61 L62 L63 L73 L84 | L51 L56 L61 L63 L66 L68 L70 L72 L81 | L51 L57 L61 L62 L63 | L63 L65 L70 L73 L84 L86 of sketch 2 contours L0 L2 L19 L41 L55 | L2 L10 L16 L17 L23 L24 L32 L33 L44 L45 | L0 L10 L41 L42 L44 L45 | L0 L3 L5 L19 L55 L56 | L0 L3 L10 L42 L45 L51 L56 | L2 L19 L28 L55 | L9 L19 L28 L55 | L2 L25 L28 L55 | L3 L4 L5 L56 | L3 L4 L5 L10 L11 L12 L28 L56 | L5 L9 L28 L56 | L9 L25 L28 L55 | L2 L9 L23 L24 L25 L26 | L9 L25 L28 L56 | L1 L16 L29 L30 L32 L33 | L13 L25 L28 L56 | L9 L13 L25 L26 | L2 L26 L27 L53 | L1 L6 L16 L30 L33 L39 L54 | L1 L2 L18 L29 L53 | L9 L26 L27 L53 | L9 L26 L27 L54 | L2 L18 L27 L53 | L1 L6 L8 L18 L53 L54 | L9 L18 L27 L53 | L8 L9 L27 L54 | L13 L26 L27 L54 | L6 L7 L8 L14 L15 L16 L27 L54 | L6 L7 L8 L54 | L63 L64 L84 L88 L90 L101 | L64 L70 L84 L86 L88 L90 L92 | L59 L63 L64 L68 L90 L95 L98 L105 L107 L108 | L60 L84 L96 L101 L105 | L60 L75 L84 L86 L92 L96 | L64 L71 L73 L75 L82 L86 L92 L93 | L60 L73 L96 L105 | L60 L73 L96 L104 | L71 L75 L86 L92 | L73 L75 L86 L104 | L73 L85 L96 L105 | L73 L85 L96 L104 | L59 L65 L68 L69 L81 L95 | L73 L85 L86 L104 | L79 L85 L98 L104 L105 L108 | L59 L65 L69 L74 L83 L95 L97 | L65 L81 L103 L105 L109 | L73 L85 L86 L110 | L79 L85 L104 L110 | L65 L76 L83 L97 L103 L109 | L66 L103 L105 L109 | L66 L79 L103 L104 | L66 L79 L97 L104 | L66 L79 L103 L105 | L66 L67 L72 L76 L83 L95 L97 L102 | L66 L103 L104 L109 | L66 L79 L97 L110 | L66 L76 L97 L104 | L67 L76 L83 L97 of sketch 3 contours L5 L11 L14 L15 L70 L71 | L3 L5 L7 L15 | L3 L4 L11 L12 L15 L55 L69 | L5 L11 L14 L16 L19 L70 L71 | L9 L10 L18 | L5 L10 L11 L18 L70 | L5 L10 L11 L16 L19 L20 L70 | L5 L14 L16 L51 L70 L71 | L4 L9 L10 L11 L55 | L4 L11 L12 L16 L55 L69 | L4 L10 L11 L16 L55 | L5 L14 L39 L51 L70 L71 | L5 L16 L20 L51 L70 L76 | L4 L12 L16 L51 L55 L69 | L10 L16 L51 L76 | L4 L10 L16 L51 L55 | L14 L23 L24 L30 L31 L32 L33 L37 L71 | L5 L14 L24 L30 L39 L70 L71 | L5 L8 L10 L51 L70 | L4 L12 L17 L39 L51 L55 L69 | L4 L5 L8 L10 L17 L39 L51 L55 L70 | L14 L23 L24 L30 L31 L37 L71 | L5 L14 L21 L24 L30 L48 L70 L71 | L4 L5 L25 L39 L55 L70 | L4 L12 L29 L39 L40 L55 L69 | L12 L28 L29 L40 L41 L42 L43 L47 L69 | L5 L14 L21 L22 L48 L70 L71 | L4 L5 L21 L25 L26 L48 L55 L70 | L4 L12 L26 L29 L40 L48 L55 L69 | L12 L28 L29 L40 L41 L47 L69 | L5 L14 L22 L38 L70 L71 | L4 L5 L21 L26 L48 L49 L55 L70 | L4 L12 L26 L27 L46 L48 L55 L69 | L5 L14 L38 L61 L70 L71 | L4 L5 L49 L54 L55 L70 | L4 L12 L27 L38 L46 L55 L69 | L5 L14 L58 L61 L70 L71 | L4 L5 L38 L54 L55 L70 | L4 L5 L38 L55 L59 L61 L64 L68 L70 | L4 L12 L38 L55 L61 L64 L69 | L5 L14 L58 L67 L70 L71 L73 | L5 L59 L61 L68 L70 | L5 L58 L59 L61 L62 L70 | L4 L12 L55 L58 L61 L69 | L5 L14 L70 L71 L72 L73 | L5 L58 L62 L65 L67 L70 L75 | L4 L55 L58 L59 L61 | L4 L12 L55 L58 L69 L73 | L4 L5 L6 L12 L13 L14 L55 L69 L70 L71 L72 | L5 L65 L70 L73 L75 | L5 L60 L70 L73 L75 | L58 L59 L63 L65 L73 L75 | L63 L65 L75 | L4 L55 L58 L59 L73 | L4 L12 L55 L69 L72 L73 | L5 L57 L70 L72 L75 | L4 L5 L6 L55 L70 L72 | L57 L60 L75 | L59 L60 L73 L75 | L4 L55 L57 L59 L73 | L4 L55 L57 L72 L75 | L57 L59 L60 L75 bodies 1
extrude "floorTolerance (1)" cut 4 faces at (150.1667, 21.5795, 2) (136.3333, 18.4205, 2) (54.8333, 18.4205, 2) (29.8333, 21.5795, 2) along direction (0, 0, 1) blind 0.7 on bodies 1 bodies 1
extrude "Extrude45" add 2 faces at (145.6667, 26.7462, 2) (33.1667, 26.7462, 2) along direction (0, 0, 1) blind 0.35 on bodies 1 bodies 1
extrude "Extrude46" cut 4 faces at (37.9167, 32.5833, 2) (30.9167, 10.6667, 2) (142.0833, 32.5833, 2) (149.0833, 11.3333, 2) along direction (0, 0, -1) blind 0.35 on bodies 2 3 bodies 3 2
extrude "pullerBottom" add sketch "puller" against normal blind 2 separate body contours L0 L2 L19 L41 L55 | L0 L3 L5 L19 L55 L56 | L2 L19 L28 L55 | L9 L19 L28 L55 | L2 L25 L28 L55 | L3 L4 L5 L56 | L9 L25 L28 L55 | L2 L9 L23 L24 L25 L26 | L2 L26 L27 L53 | L1 L2 L18 L29 L53 | L9 L26 L27 L53 | L2 L18 L27 L53 | L1 L6 L8 L18 L53 L54 | L9 L18 L27 L53 | L6 L7 L8 L54 makes body 4
extrude "Extrude39" add sketch "puller" against normal blind 2 separate body contours L60 L84 L96 L101 L105 | L60 L75 L84 L86 L92 L96 | L60 L73 L96 L105 | L60 L73 L96 L104 | L71 L75 L86 L92 | L73 L85 L96 L105 | L73 L85 L96 L104 | L79 L85 L98 L104 L105 L108 | L65 L81 L103 L105 L109 | L65 L76 L83 L97 L103 L109 | L66 L103 L105 L109 | L66 L79 L103 L104 | L66 L79 L103 L105 | L66 L103 L104 L109 | L67 L76 L83 L97 makes body 5
extrude "Extrude32" cut sketch "puller" against normal blind 0.7 contours L0 L3 L5 L19 L55 L56 | L9 L19 L28 L55 | L3 L4 L5 L56 | L9 L25 L28 L55 | L9 L26 L27 L53 | L1 L6 L8 L18 L53 L54 | L9 L18 L27 L53 | L6 L7 L8 L54 bodies 4
extrude "Extrude40" cut sketch "puller" against normal blind 0.7 contours L60 L75 L84 L86 L92 L96 | L60 L73 L96 L104 | L71 L75 L86 L92 | L73 L85 L96 L104 | L65 L76 L83 L97 L103 L109 | L66 L79 L103 L104 | L66 L103 L104 L109 | L67 L76 L83 L97 bodies 5
extrude "pullerTop" add sketch "puller" along normal blind 4.7 contours L0 L2 L19 L41 L55 | L0 L10 L41 L42 L44 L45 | L2 L19 L28 L55 | L10 L42 L43 L44 L45 | L2 L25 L28 L55 | L2 L9 L23 L24 L25 L26 | L16 L30 L31 L32 L33 | L1 L16 L29 L30 L32 L33 | L2 L26 L27 L53 | L1 L2 L18 L29 L53 | L2 L18 L27 L53 bodies 4
extrude "Extrude41" add sketch "puller" along normal blind 4 contours L58 L63 L64 L88 L90 | L63 L64 L84 L88 L90 L101 | L60 L84 L96 L101 L105 | L60 L73 L96 L105 | L73 L85 L96 L105 | L59 L65 L68 L69 L81 L95 | L59 L61 L68 L69 L95 | L79 L85 L98 L104 L105 L108 | L65 L81 L103 L105 L109 | L66 L103 L105 L109 | L66 L79 L103 L105 bodies 5
extrude "slide (1)" add sketch "slide" against normal blind 2 separate body contours L4 L5 L7 L9 L55 L70 | L9 L10 L18 | L4 L9 L10 L11 L55 | L4 L10 L11 L16 L55 | L4 L10 L16 L51 L55 | L4 L5 L8 L10 L17 L39 L51 L55 L70 | L4 L5 L25 L39 L55 L70 | L4 L5 L21 L25 L26 L48 L55 L70 | L4 L5 L21 L26 L48 L49 L55 L70 | L4 L5 L49 L54 L55 L70 | L4 L5 L38 L54 L55 L70 | L4 L5 L38 L55 L59 L61 L64 L68 L70 | L4 L55 L58 L59 L61 | L4 L55 L58 L59 L73 | L5 L57 L70 L72 L75 | L4 L5 L6 L55 L70 L72 | L57 L60 L75 | L4 L55 L57 L59 L73 | L4 L55 L57 L72 L75 | L57 L59 L60 L75 makes body 6
extrude "Extrude17" add sketch "slide" along normal blind 1.3 contours L14 L23 L24 L30 L31 L37 L71 | L5 L14 L21 L24 L30 L48 L70 L71 | L14 L22 L31 L36 L71 | L5 L14 L21 L22 L48 L70 L71 | L4 L5 L21 L25 L26 L48 L55 L70 | L4 L12 L26 L29 L40 L48 L55 L69 | L12 L28 L29 L40 L41 L47 L69 | L22 L23 L31 L36 L37 | L4 L5 L21 L26 L48 L49 L55 L70 | L4 L12 L26 L27 L46 L48 L55 L69 | L12 L27 L28 L41 L46 L47 L69 bodies 6
sketch "hookBase" plane through (0, 0, 0) normal (0, 0, -1) x (1, 0, 0)
  circle A0 centre (176.25, -22.3937) radius 1.5
  circle A1 centre (145.75, -22.3937) radius 1.5
  line L0 (25.5, -24.4885) -> (174.5, -24.4885)
  line L1 (32.5, -15.5115) -> (25.5, -15.5115)
  line L2 (90, -40) -> (90, 0)
  line L3 (100, -24.4885) -> (100.0511, -15.4143)
  circle A2 centre (54.2765, -21.879) radius 1.5
  circle A3 centre (3.75, -22.3937) radius 1.5
  line L4 (25.5, -15.5115) -> (25.5, -24.4885)
  line L5 (34.75, -17.7615) -> (32.5, -15.5115)
  line L6 (174.5, -24.4885) -> (174.5, -15.5115)
  line L7 (174.5, -15.5115) -> (167.5, -15.5115)
  line L8 (167.5, -15.5115) -> (165.25, -17.7615)
  line L9 (165.25, -17.7615) -> (144, -17.7615)
  line L10 (144, -17.7615) -> (144, -15.5115)
  line L11 (56, -15.5115) -> (56, -17.7615)
  line L12 (56, -17.7615) -> (34.75, -17.7615)
  line L13 (0, 0) -> (0, -40)
  line L14 (0, -40) -> (180, -40)
  line L15 (180, -40) -> (180, 0)
  line L16 (180, 0) -> (0, 0)
  line L17 (140.5, -33.5) -> (140.5, -27.75)
  line L18 (140.5, -27.75) -> (148, -27.75)
  line L19 (148, -27.75) -> (148, -33.5)
  line L20 (148, -33.5) -> (154.5, -33.5)
  line L21 (154.5, -33.5) -> (154.5, -24.7385)
  line L22 (154.5, -24.7385) -> (120, -24.7385)
  line L23 (120, -24.7385) -> (120, -27.7385)
  line L24 (120, -27.7385) -> (116.5, -27.7385)
  line L25 (116.5, -27.7385) -> (116.5, -24.7385)
  line L26 (116.5, -24.7385) -> (25.5, -24.7385)
  line L27 (25.5, -24.7385) -> (25.5, -33.5)
  line L28 (25.5, -33.5) -> (32, -33.5)
  line L29 (32, -33.5) -> (32, -27.75)
  line L30 (32, -27.75) -> (39.5, -27.75)
  line L31 (39.5, -27.75) -> (39.5, -33.5)
  line L32 (39.5, -33.5) -> (50.5, -33.5)
  line L33 (50.5, -33.5) -> (50.5, -36.5)
  line L34 (50.5, -36.5) -> (2, -36.5)
  line L35 (2, -36.5) -> (2, -3.5)
  line L36 (2, -3.5) -> (50.5, -3.5)
  line L37 (50.5, -3.5) -> (50.5, -6.5)
  line L38 (50.5, -6.5) -> (35.5, -6.5)
  line L39 (35.5, -15.2615) -> (116.5, -15.2615)
  line L40 (116.5, -15.2615) -> (116.5, -12.2615)
  line L41 (116.5, -12.2615) -> (120, -12.2615)
  line L42 (120, -12.2615) -> (120, -15.2615)
  line L43 (120, -15.2615) -> (144.5, -15.2615)
  line L44 (144.5, -15.2615) -> (144.5, -6.5)
  line L45 (144.5, -6.5) -> (129.5, -6.5)
  line L46 (129.5, -6.5) -> (129.5, -3.5)
  line L47 (129.5, -3.5) -> (178, -3.5)
  line L48 (178, -3.5) -> (178, -36.5)
  line L49 (178, -36.5) -> (129.5, -36.5)
  line L50 (129.5, -36.5) -> (129.5, -33.5)
  line L51 (129.5, -33.5) -> (140.5, -33.5)
  line L52 (145.75, -22.3937) -> (176.25, -22.3937)
  line L53 (144, -15.5115) -> (56, -15.5115)
  line L54 (35.5, -6.5) -> (35.5, -15.2615)
  dimension "d107" = 3
  dimension "d109" = 3
  dimension "d305" = 3.75
  dimension "d306" = 30.5
  constraint midpoint L0 L3.start
  constraint symmetric A1 L3 A2
  constraint symmetric A0 L2 A3
  constraint midpoint L2.end L16
  constraint midpoint L2.start L14
  constraint coincident A1.centre L52.start
  constraint coincident A0.centre L52.end
  constraint perpendicular L6 L52
  measures "d107" diameter of A0
  measures "d109" diameter of A1
  measures "d305" distance of A0.centre L15
  measures "d306" distance of A1.centre A0.centre
extrude "Extrude12" add sketch "hookBase" along normal blind 2 contours A0 | A1 | A2 | A3 bodies 4 5 6
sketch "hookSlot" plane through (0, 0, -2) normal (0, 0, -1) x (1, 0, 0)
  circle A0 centre (145.75, -22.3937) radius 1.5
  line L0 (176.25, -22.3937) -> (145.75, -22.3937)
  circle A1 centre (176, -22.3937) radius 1.25
  circle A2 centre (146, -22.3937) radius 1.25
  line L1 (25.5, -24.4885) -> (174.5, -24.4885)
  line L2 (32.5, -15.5115) -> (25.5, -15.5115)
  line L3 (0, 0) -> (0, -40)
  line L4 (0, -40) -> (180, -40)
  line L5 (180, -40) -> (180, 0)
  line L6 (180, 0) -> (0, 0)
  line L7 (140.5, -33.5) -> (140.5, -27.75)
  line L8 (140.5, -27.75) -> (148, -27.75)
  line L9 (154.5, -33.5) -> (154.5, -24.7385)
  line L10 (154.5, -24.7385) -> (120, -24.7385)
  line L11 (120, -24.7385) -> (120, -27.7385)
  line L12 (120, -27.7385) -> (116.5, -27.7385)
  line L13 (116.5, -27.7385) -> (116.5, -24.7385)
  line L14 (116.5, -24.7385) -> (25.5, -24.7385)
  line L15 (25.5, -24.7385) -> (25.5, -33.5)
  line L16 (32, -27.75) -> (39.5, -27.75)
  line L17 (39.5, -27.75) -> (39.5, -33.5)
  line L18 (25.5, -33.5) -> (32, -33.5)
  line L19 (50.5, -33.5) -> (50.5, -36.5)
  line L20 (50.5, -36.5) -> (2, -36.5)
  line L21 (2, -36.5) -> (2, -3.5)
  line L22 (2, -3.5) -> (50.5, -3.5)
  line L23 (50.5, -3.5) -> (50.5, -6.5)
  line L24 (50.5, -6.5) -> (35.5, -6.5)
  line L25 (35.5, -15.2615) -> (116.5, -15.2615)
  line L26 (116.5, -15.2615) -> (116.5, -12.2615)
  line L27 (116.5, -12.2615) -> (120, -12.2615)
  line L28 (120, -12.2615) -> (120, -15.2615)
  line L29 (120, -15.2615) -> (144.5, -15.2615)
  line L30 (144.5, -6.5) -> (129.5, -6.5)
  line L31 (129.5, -6.5) -> (129.5, -3.5)
  line L32 (129.5, -3.5) -> (178, -3.5)
  line L33 (178, -3.5) -> (178, -36.5)
  line L34 (178, -36.5) -> (129.5, -36.5)
  line L35 (129.5, -36.5) -> (129.5, -33.5)
  line L36 (129.5, -33.5) -> (140.5, -33.5)
  line L37 (100, -24.4885) -> (100, -15.0887)
  line L38 (90, -40) -> (90, 0)
  circle A3 centre (54, -22.3937) radius 1.25
  circle A4 centre (4, -22.3937) radius 1.25
  line L39 (144.5, -15.2615) -> (144.5, -6.5)
  circle A5 centre (145.75, -22.3937) radius 1.5
  line L40 (25.5, -15.5115) -> (25.5, -24.4885)
  line L41 (148, -27.75) -> (148, -33.5)
  line L42 (32, -33.5) -> (32, -27.75)
  circle A6 centre (54.2765, -21.879) radius 1.5
  circle A7 centre (176.25, -22.3937) radius 1.5
  circle A8 centre (3.75, -22.3937) radius 1.5
  line L43 (34.75, -17.7615) -> (32.5, -15.5115)
  line L44 (174.5, -24.4885) -> (174.5, -15.5115)
  line L45 (174.5, -15.5115) -> (167.5, -15.5115)
  line L46 (167.5, -15.5115) -> (165.25, -17.7615)
  line L47 (165.25, -17.7615) -> (144, -17.7615)
  line L48 (144, -17.7615) -> (144, -15.5115)
  line L49 (56, -15.5115) -> (56, -17.7615)
  line L50 (56, -17.7615) -> (34.75, -17.7615)
  line L51 (144, -15.5115) -> (56, -15.5115)
  line L52 (148, -33.5) -> (154.5, -33.5)
  line L53 (39.5, -33.5) -> (50.5, -33.5)
  line L54 (35.5, -6.5) -> (35.5, -15.2615)
  point P0 (146, -22.3937)
  point P1 (176, -22.3937)
  dimension "d126" = 0.25
  dimension "d127" = 0.25
  dimension "d128" = 2.5
  dimension "d129" = 2.5
  constraint coincident L0 P0
  constraint coincident L0 P1
  constraint coincident P1 A1.centre
  constraint coincident P0 A2.centre
  constraint midpoint L1 L37.start
  constraint midpoint L4 L38.start
  constraint midpoint L6 L38.end
  constraint symmetric A2 L37 A3
  constraint symmetric A1 L38 A4
  constraint coincident L0.start A7.centre
  constraint coincident A0.centre L0.end
  constraint perpendicular L1 L37
  measures "d126" distance of A0.centre P0
  measures "d127" distance of L0.start P1
  measures "d128" diameter of A1
  measures "d129" diameter of A2
extrude "Extrude14" add sketch "hookSlot" along normal blind 0.5 contours A2 | A1 | A3 A6 | A3 A6 | A4 picked at (53.9337, -22.5762) picked at (53.5152, -23.2962) bodies 4 5 6